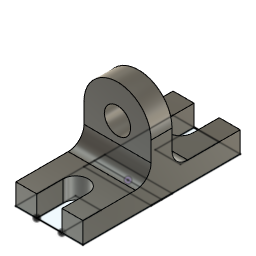
Exercise_4 v1 (Autodesk Fusion 360 design; units mm, degrees)
Autodesk Fusion 360 part; units mm, degrees
sketch "Sketch1" plane through (0, 0, 0) normal (0, 0, 1) x (1, 0, 0)
  line L0 (-32, 75) -> (32, 75)
  line L1 (32, 75) -> (32, -75)
  line L2 (32, -75) -> (-32, -75)
  line L3 (-32, -75) -> (-32, 75)
  line L4 (-32, -10) -> (32, -10)
  line L5 (32, -10) -> (32, 10)
  line L6 (32, 10) -> (-32, 10)
  line L7 (-32, 10) -> (-32, -10)
  line L8 (-12, 75) -> (12, 75)
  line L9 (12, 75) -> (12, 38)
  line L10 (12, 38) -> (-12, 38)
  line L11 (-12, 38) -> (-12, 75)
  line L12 (-32, 0) -> (32, 0)
  line L13 (-12, -38) -> (-12, -75)
  line L14 (12, -38) -> (-12, -38)
  line L15 (12, -75) -> (12, -38)
  dimension "d1" = 64
  dimension "d2" = 150
  dimension "d3" = 75
  dimension "d4" = 32
  dimension "d5" = 20
  dimension "d6" = 10
  dimension "d7" = 24
  dimension "d8" = 37
  dimension "d9" = 12
  constraint horizontal L0
  constraint vertical L1
  constraint horizontal L2
  constraint vertical L3
  constraint horizontal L4
  constraint vertical L5
  constraint horizontal L6
  constraint vertical L7
  constraint coincident L1 L5.end
  constraint coincident L3 L4.start
  constraint horizontal L8
  constraint vertical L9
  constraint horizontal L10
  constraint vertical L11
  constraint coincident L0 L8.start
  constraint midpoint L7 L12.start
  constraint midpoint L1 L12.end
  constraint symmetric L8.start L12 L13.end
  constraint symmetric L8.end L12 L15.start
  constraint symmetric L9.end L12 L14.start
  constraint symmetric L10.end L12 L13.start
  measures "d1" distance of L0.start L0.end
  measures "d2" distance of L0.end L1.end
  measures "d3" distance of origin L0
  measures "d4" distance of origin L1
  measures "d5" distance of L4.start L6.end
  measures "d6" distance of origin L4
  measures "d7" distance of L8.start L8.end
  measures "d8" distance of L8.start L10.end
  measures "d9" distance of origin L11
extrude "Extrude1" add sketch "Sketch1" along normal blind 20 contours L0 L1 L3 L6 L9 L10 L11 | L1 L2 L3 L4 L13 L14 L15 makes body 1 at (-4, -19.3333, 0) makes body 2 at (4, 19.3333, 0)
extrude "Extrude2" add sketch "Sketch1" along normal blind 86 contours L1 L3 L5 L6 L7 L12 | L1 L3 L4 L5 L7 L12 bodies 1 2
sketch "Sketch2" plane through (0, -10, 0) normal (0, -1, 0) x (1, 0, 0)
  line L0 (-32, 20) -> (32, 20)
  line L1 (32, 20) -> (32, 86)
  line L2 (32, 86) -> (-32, 86)
  line L3 (-32, 86) -> (-32, 20)
  circle A0 centre (0, 54) radius 12.5
  line L4 (32, 0) -> (-32, 0)
  dimension "d14" = 25
  dimension "d16" = 54
  measures "d14" diameter of A0
  measures "d16" distance of A0.centre L4
extrude "Extrude3" cut sketch "Sketch2" against normal up to surface (20 mm away) contours A0 bodies 1
fillet "Fillet1" radius 32 2 edges at (32, 0, 86) (-32, 0, 86) on bodies 1
fillet "Fillet2" radius 15 2 edges at (0, 10, 20) (0, -10, 20) on bodies 1
fillet "Fillet3" radius 12 4 edges at (-12, -38, 10) (12, -38, 10) (12, 38, 10) (-12, 38, 10) on bodies 1
equation "d1 = ( 2 * 20 ) * 1 mm + 24 mm"
equation "d2 = ( 2 * 65 ) * 1 mm + 20 mm"
equation "d3 = ( 150 / 2 ) * 1 mm"
equation "d8 = 25 mm + 12 mm"
equation "d12 = 54 mm + 32 mm"
